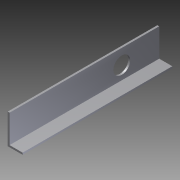
# Autodesk Inventor part: 8 ball bearing plate right
Saved by Autodesk Inventor 2012 (Build 160160000, 160)
## iProperties
Created: 2013-09-05
Part Number: 8 ball bearing plate right
Material: Default
Document SubType Name: Modeling
Designer: Bryce
Density: 1 g/cm^3
Author: Bryce
Autodesk Inventor part; units mm, degrees
ref_plane "YZ Plane" through (0, 0, 0) normal (1, 0, 0) x (0, 1, 0)
ref_plane "XZ Plane" through (0, 0, 0) normal (0, 1, 0) x (-1, 0, 0)
ref_plane "XY Plane" through (0, 0, 0) normal (0, 0, 1) x (1, 0, 0)
sketch "Sketch1" plane through (0, 0, 0) normal (0, 0, 1) x (1, 0, 0)
  line L0 (0, 0) -> (25.4, 0)
  line L1 (25.4, 0) -> (25.4, 3.175)
  line L2 (3.175, 50.8) -> (0, 50.8)
  line L3 (0, 50.8) -> (0, 0)
  line L4 (3.175, 50.8) -> (3.175, 3.175)
  line L5 (3.175, 3.175) -> (25.4, 3.175)
  dimension "d0" = 50.8
  dimension "d1" = 25.4
  dimension "d2" = 3.175
  dimension "d3" = 3.175
  constraints: 12 end point, 2 parallel, 1 horizontal, 1 perpendicular
  measures "d0" distance of L2.end L0.start
  measures "d1" distance of L0.start L0.end
  measures "d2" distance between parallel lines of L0 L5
  measures "d3" distance between parallel lines of L3 L4
extrude "Extrusion1" add sketch "Sketch1" along normal blind 254
sketch "Sketch2" plane through (0, 0, 0) normal (-1, 0, 0) x (0, 0, 1)
  line L0 (0, 50.8) -> (0, 0) projected
  line L1 (0, 0) -> (254, 0) projected
  circle A0 centre (63.5, 25.4) radius 14.2875
  dimension "d6" = 28.575
  dimension "d7" = 63.5
  dimension "d8" = 25.4
  constraints: 1 centre point
  measures "d6" diameter of A0
  measures "d7" distance from line of L0 A0.centre
  measures "d8" distance from line of L1 A0.centre
extrude "Extrusion2" cut sketch "Sketch2" against normal through all
equation "\"d2\" = d3"
body "Solid1"
